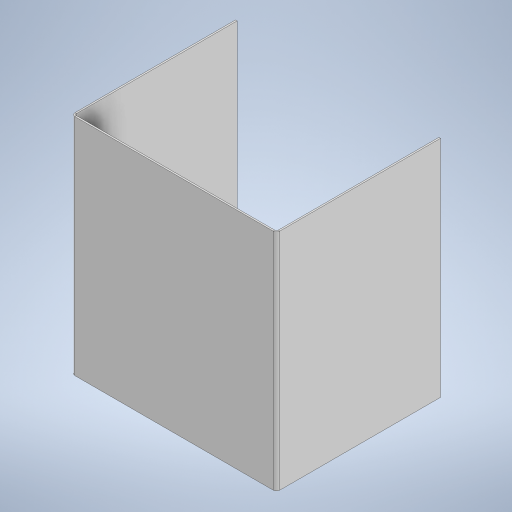
# Autodesk Inventor part: Part1
Saved by Autodesk Inventor 2023 (Build 270158000, 158)
## iProperties
Created: 2023-03-06
Part Number: Part1
Material: Generic
Document SubType Name: Sheet Metal
Designer: ACER
Density: 1 g/cm^3
Sheet Metal Rule: Default_mm
Appearance: Default
Flat Pattern Width: 27.3564 cm
Flat Pattern Length: 64.3048 cm
Flat Pattern Area: 1759.15 cm^2
Sheet Metal Width: 273.564 mm
Sheet Metal Length: 643.048 mm
Sheet Metal Area: 175914.762 mm^2
Author: ACER
Autodesk Inventor part; units mm, degrees
ref_plane "YZ Plane" through (0, 0, 0) normal (1, 0, 0) x (0, 1, 0)
ref_plane "XZ Plane" through (0, 0, 0) normal (0, 1, 0) x (-1, 0, 0)
ref_plane "XY Plane" through (0, 0, 0) normal (0, 0, 1) x (1, 0, 0)
sketch "Sketch1" plane through (0, 0, 0) normal (0, 0, 1) x (1, 0, 0)
  line L0 (125, -136.782) -> (-125, -136.782)
  line L1 (-125, -136.782) -> (-125, 136.782)
  line L2 (-125, 136.782) -> (125, 136.782)
  line L3 (125, 136.782) -> (125, -136.782)
  line L4 (125, -136.782) -> (-125, 136.782) construction
  line L5 (-125, -136.782) -> (125, 136.782) construction
  point P0 (0, 0)
  dimension "d1" = 250
  measures "d1" distance of L1.end L2.end
extrude "Plate1" add sketch "Sketch1" along normal blind 2
sketch "Sketch2" plane through (123, -136.782, 2) normal (1, 0, 0) x (0, 1, 0)
  line L0 (273.5641, 0) -> (0, 0)
  line L1 (0, 0) -> (0, -200)
  line L2 (0, -200) -> (273.5641, -200)
  line L3 (273.5641, -200) -> (273.5641, 0)
  constraints: 6 end point, 1 horizontal, 1 perpendicular, 1 vertical
edge flange "Flange1" height 200 angle 90 thickness 2 bend radius 2 thickness toward (1, 0, 0) relief tear relief width 2 relief depth 1 edges at (125, 0, 0) wall of the first edge with corners at (123, 136.782, 2) (123, -136.782, 2) (123, -136.782, -198) (123, 136.782, -198)
bend "Bend1"
corner "Corner1"
sketch "Sketch3" plane through (-123, 136.782, 2) normal (-1, 0, 0) x (0, -1, 0)
  line L0 (273.5641, 0) -> (0, 0)
  line L1 (0, 0) -> (0, -200)
  line L2 (0, -200) -> (273.5641, -200)
  line L3 (273.5641, -200) -> (273.5641, 0)
  constraints: 6 end point, 1 horizontal, 1 perpendicular, 1 vertical
edge flange "Flange2" height 200 angle 90 thickness 2 bend radius 2 thickness toward (-1, 0, 0) relief tear relief width 2 relief depth 1 edges at (-125, 0, 0) wall of the first edge with corners at (-123, -136.782, 2) (-123, 136.782, 2) (-123, 136.782, -198) (-123, -136.782, -198)
bend "Bend2"
corner "Corner2"
equation "\"d0\" = Thickness"
equation "\"d2\" = BendReliefWidth"
equation "\"d3\" = BendReliefDepth"
equation "\"d4\" = MinimumRemnant"
equation "\"d5\" = TransitionRadius"
equation "\"d8\" = BendRadius"
equation "\"d9\" = CornerReliefSize"
equation "\"d10\" = GapSize"
equation "\"d11\" = JacobiRadiusSize"
equation "\"d12\" = BendReliefWidth"
equation "\"d13\" = BendReliefDepth"
equation "\"d14\" = MinimumRemnant"
equation "\"d15\" = TransitionRadius"
equation "\"d18\" = BendRadius"
equation "\"d19\" = CornerReliefSize"
equation "\"d20\" = GapSize"
equation "\"d21\" = JacobiRadiusSize"
equation "\"BendRadius\" = Thickness"
equation "\"BendReliefWidth\" = Thickness"
equation "\"BendReliefDepth\" = 0.5 * Thickness"
equation "\"CornerReliefSize\" = 4 * Thickness"
equation "\"MinimumRemnant\" = 2 * Thickness"
equation "\"TransitionRadius\" = BendRadius"
equation "\"JacobiRadiusSize\" = BendRadius"
equation "\"GapSize\" = Thickness"
equation "\"Thickness\" = 2"
body "Solid1"
